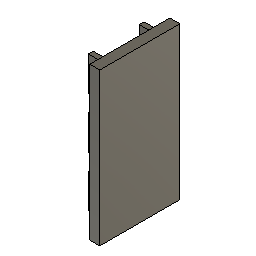
slot_gauge (Autodesk Fusion 360 design; units mm, degrees)
part number: 2026-09-02-15-09-24-795
Autodesk Fusion 360 part; units mm, degrees
sketch "Gauge plate" plane through (0, 0, 0) normal (0, 1, 0) x (1, 0, 0)
  line L0 (0, 0) -> (5, 0)
  line L1 (5, 0) -> (5, -76)
  line L2 (5, -76) -> (0, -76)
  line L3 (0, -76) -> (0, 0)
extrude "Gauge plate (1)" add sketch "Gauge plate" along normal mid plane 40
sketch "Hook profiles" plane through (0, 0, 0) normal (0, 1, 0) x (1, 0, 0)
  line L0 (0, -74) -> (-6.8, -74)
  line L1 (-6.8, -74) -> (-6.8, -57)
  line L2 (-6.8, -57) -> (-2.8, -57)
  line L3 (-2.8, -57) -> (-2.8, -69)
  line L4 (-2.8, -69) -> (0, -69)
  line L5 (0, -69) -> (0, -74)
  line L6 (0, -48.6) -> (-6.8, -48.6)
  line L7 (-6.8, -48.6) -> (-6.8, -31.6)
  line L8 (-6.8, -31.6) -> (-2.8, -31.6)
  line L9 (-2.8, -31.6) -> (-2.8, -43.6)
  line L10 (-2.8, -43.6) -> (0, -43.6)
  line L11 (0, -43.6) -> (0, -48.6)
  line L12 (0, -23.2) -> (-6.8, -23.2)
  line L13 (-6.8, -23.2) -> (-6.8, -6.2)
  line L14 (-6.8, -6.2) -> (-2.8, -6.2)
  line L15 (-2.8, -6.2) -> (-2.8, -18.2)
  line L16 (-2.8, -18.2) -> (0, -18.2)
  line L17 (0, -18.2) -> (0, -23.2)
extrude "Hook slab" add sketch "Hook profiles" along normal mid plane 27.8
extrude "Hook column split" cut sketch "Hook profiles" along normal mid plane 23
named bodies: "slot_gauge"
